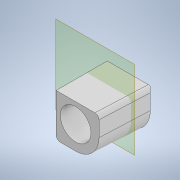
# Autodesk Inventor part: CornerHolder
Saved by Autodesk Inventor 2022 (Build 260153000, 153)
## iProperties
Created: 2021-04-22
Part Number: CornerHolder
Material: Generic
Document SubType Name: Modeling
Designer: Viktor
Density: 1 g/cm^3
Appearance: Default
Author: Viktor
## iProperties of the stored document CornerHolder_3DPrint.ipt
Created: 2021-04-22
Part Number: CornerHolder_3DPrint
Material: Generic
Document SubType Name: Modeling
Designer: Viktor
Density: 1 g/cm^3
Appearance: Default
Author: Viktor
Autodesk Inventor part; units mm, degrees
ref_plane "YZ Plane" through (0, 0, 0) normal (1, 0, 0) x (0, 1, 0)
ref_plane "XZ Plane" through (0, 0, 0) normal (0, 1, 0) x (-1, 0, 0)
ref_plane "XY Plane" through (0, 0, 0) normal (0, 0, 1) x (1, 0, 0)
sketch "Sketch1" plane through (0, 0, 0) normal (0, 0, 1) x (1, 0, 0)
  circle A0 centre (0, 0) radius 12.5
  line L0 (12.5, 0) -> (12.5, 22.5)
  line L1 (12.5, 22.5) -> (-22.5, 22.5)
  line L2 (-22.5, 22.5) -> (-22.5, -12.5)
  line L3 (-22.5, -12.5) -> (0, -12.5)
  dimension "d0" = 25
  dimension "d1" = 35
  dimension "d2" = 35
  constraints: 8 end point, 3 perpendicular, 2 point on circle, 1 centre point, 1 coincident, 1 vertical
  measures "d0" diameter of A0
  measures "d1" distance between parallel lines of L3 L1
  measures "d2" distance between parallel lines of L0 L2
extrude "Extrusion1" add sketch "Sketch1" along normal blind 25
draft "FaceDraft1" angle 2.5 pull direction (0, 0, 1) faces at (-15, -12.5, 8.3333) (3.6844, -11.9447, 16.6667) (12.5, 7.5, 8.3333) fixed edges at (-11.25, -12.5, 0) (8.8388, -8.8388, 0) (12.5, 11.25, 0)
sketch "Sketch2" plane through (0, 0, 0) normal (0, 0, -1) x (-1, 0, 0)
  circle A0 centre (0, 0) radius 2.75
  dimension "d6" = 5.5
  constraints: 1 centre point, 1 coincident
  measures "d6" diameter of A0
extrude "Extrusion2" cut sketch "Sketch2" against normal through all
ref_plane "Work Plane1" through (0, 0, 10) normal (0, 0, -1) x (-1, 0, 0)
sketch "Sketch3" plane through (0, 0, 25) normal (0, 0, 1) x (1, 0, 0)
  circle A0 centre (0, 0) radius 2.75 projected
  circle A1 centre (0, 0) radius 7.5
  dimension "d10" = 15
  constraints: 1 centre point, 1 coincident
  measures "d10" diameter of A1
extrude "Extrusion3" cut sketch "Sketch3" against normal up to surface (15 mm away)
chamfer "Chamfer1" distance 1 angle 45 6 edges at (8.8388, -8.8388, 0) (12.5, 11.25, 0) (-11.25, -12.5, 0) (2.75, 0, 0) (-5, 22.5, 0) (-22.5, 5, 0)
sketch "Sketch4" plane through (0, 0, 25) normal (0, 0, 1) x (1, 0, 0)
  line L0 (12.4564, 22.499) -> (12.4564, 0) projected
  line L1 (0, -12.4564) -> (-22.499, -12.4564) projected
  line L2 (12.4564, 9.5436) -> (-9.5436, 9.5436)
  line L3 (-9.5436, -12.4564) -> (-9.5436, 9.5436)
  arc A0 (0, -12.4564) -> (12.4564, 0) centre (0, 0) ccw projected
  line L4 (22, -23) -> (-37, -23)
  line L5 (-37, -23) -> (-37, 27)
  line L6 (-37, 27) -> (22, 27)
  line L7 (22, 27) -> (22, -23)
  point P0 (0, 0)
  dimension "d16" = 22
  dimension "d17" = 22
  constraints: 12 end point, 2 horizontal, 2 parallel, 2 point on line, 1 perpendicular, 1 vertical
  measures "d16" distance between parallel lines of L0 L3
  measures "d17" distance between parallel lines of L1 L2
extrude "Extrusion4" cut sketch "Sketch4" against normal through all
fillet "Fillet1" radius 2 2 edges at (-9.5436, -11.9324, 12.9995) (11.9324, 9.5436, 12.9995)
equation "\"d2\" = d1"
equation "\"d17\" = d16"
body "Solid1"
